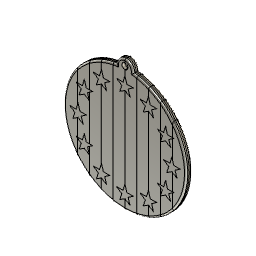
EU-Ohrring-Volt-v4 (Autodesk Fusion 360 design; units mm, degrees)
Autodesk Fusion 360 part; units mm, degrees
sketch "Skizze1" plane through (0, 0, 0) normal (0, 1, 0) x (1, 0, 0)
  circle A0 centre (0, 0) radius 15
  dimension "d1" = 30
  constraint coincident A0.centre origin
  measures "d1" diameter of A0
extrude "Extrusion1" add sketch "Skizze1" along normal blind 1.5 makes body 1
sketch "Skizze2" plane through (0, 0, 0) normal (0, -1, 0) x (1, 0, 0)
  circle A0 centre (0, 0) radius 15
  line L0 (2.7093, -1.1001) -> (1.6674, -1.1001)
  line L1 (1.6674, -1.1001) -> (1.3547, -0.0582)
  line L2 (1.3547, -0.0582) -> (1.0419, -1.1001)
  line L3 (1.0419, -1.1001) -> (0, -1.1001)
  line L4 (0, -1.1001) -> (0.8334, -1.6732)
  line L5 (0.8334, -1.6732) -> (0.5212, -2.6633)
  line L6 (0.5212, -2.6633) -> (1.3547, -2.1421)
  line L7 (1.3547, -2.1421) -> (2.1881, -2.6633)
  line L8 (2.1881, -2.6633) -> (1.8759, -1.6732)
  line L9 (1.8759, -1.6732) -> (2.7093, -1.1001)
extrude "Extrusion2" add sketch "Skizze2" against normal blind 0.6 separate body contours L0 L1 L2 L3 L4 L5 L6 L7 L8 L9 makes body 2
sketch "Skizze3" plane through (0, 0, 0) normal (0, 1, 0) x (1, 0, 0)
  point P0 (0, -11.5)
  point P1 (5.75, -9.9593)
  point P2 (9.9593, -5.75)
  point P3 (11.5, 0)
  point P4 (9.9593, 5.75)
  point P5 (5.75, 9.9593)
  point P6 (0, 11.5)
  point P7 (-5.75, 9.9593)
  point P8 (-9.9593, 5.75)
  point P9 (-11.5, 0)
  point P10 (-9.9593, -5.75)
  point P11 (-5.75, -9.9593)
  dimension "d9" = 360
copy_body "Körper kopieren/einfügen1" bodies 2 makes body 3
move_body "Verschieben2" bodies 3 to x (1, 0, 0) y (0, 1, 0) z (0, 0, 1) at (-1.3547, 0, 12.8608)
copy_body "Körper kopieren/einfügen2" bodies 2 makes body 4
move_body "Verschieben3" bodies 4 to x (1, 0, 0) y (0, 1, 0) z (0, 0, 1) at (4.3953, 0, 11.32)
copy_body "Körper kopieren/einfügen3" bodies 2 makes body 5
move_body "Verschieben4" bodies 5 to x (1, 0, 0) y (0, 1, 0) z (0, 0, 1) at (8.6046, 0, 7.1108)
copy_body "Körper kopieren/einfügen4" bodies 2 makes body 6
move_body "Verschieben5" bodies 6 to x (1, 0, 0) y (0, 1, 0) z (0, 0, 1) at (10.1453, 0, 1.3608)
copy_body "Körper kopieren/einfügen5" bodies 2 makes body 7
move_body "Verschieben6" bodies 7 to x (1, 0, 0) y (0, 1, 0) z (0, 0, 1) at (8.6046, 0, -4.3892)
copy_body "Körper kopieren/einfügen6" bodies 2 makes body 8
move_body "Verschieben7" bodies 8 to x (1, 0, 0) y (0, 1, 0) z (0, 0, 1) at (4.3953, 0, -8.5985)
copy_body "Körper kopieren/einfügen7" bodies 2 makes body 9
move_body "Verschieben8" bodies 9 to x (1, 0, 0) y (0, 1, 0) z (0, 0, 1) at (-1.3547, 0, -10.1392)
copy_body "Körper kopieren/einfügen8" bodies 2 makes body 10
move_body "Verschieben9" bodies 10 to x (1, 0, 0) y (0, 1, 0) z (0, 0, 1) at (-7.1047, 0, -8.5985)
copy_body "Körper kopieren/einfügen9" bodies 2 makes body 11
move_body "Verschieben10" bodies 11 to x (1, 0, 0) y (0, 1, 0) z (0, 0, 1) at (-11.314, 0, -4.3892)
copy_body "Körper kopieren/einfügen10" bodies 2 makes body 12
move_body "Verschieben11" bodies 12 to x (1, 0, 0) y (0, 1, 0) z (0, 0, 1) at (-12.8547, 0, 1.3608)
copy_body "Körper kopieren/einfügen11" bodies 2 makes body 13
move_body "Verschieben12" bodies 13 to x (1, 0, 0) y (0, 1, 0) z (0, 0, 1) at (-11.314, 0, 7.1108)
move_body "Verschieben13" bodies 2 to x (1, 0, 0) y (0, 1, 0) z (0, 0, 1) at (-7.1047, 0, 11.32)
scale "Maßstab1" factors (1.5, 1, 1.5) about (-6.0627, 0, 10.2199) bodies 2
scale "Maßstab2" factors (1.5, 1, 1.5) about (-0.3127, 0, 11.7606) bodies 3
scale "Maßstab3" factors (1.5, 1, 1.5) about (6.0627, 0, 10.2199) bodies 4
scale "Maßstab4" factors (1.5, 1, 1.5) about (10.272, 0, 6.0106) bodies 5
scale "Maßstab5" factors (1.5, 1, 1.5) about (11.8127, 0, 0.2606) bodies 6
scale "Maßstab6" factors (1.5, 1, 1.5) about (10.272, 0, -5.4894) bodies 7
scale "Maßstab7" factors (1.5, 1, 1.5) about (6.0627, 0, -9.6987) bodies 8
scale "Maßstab8" factors (1.5, 1, 1.5) about (-0.3127, 0, -11.2394) bodies 9
scale "Maßstab9" factors (1.5, 1, 1.5) about (-6.0627, 0, -9.6987) bodies 10
scale "Maßstab10" factors (1.5, 1, 1.5) about (-10.272, 0, -5.4894) bodies 11
scale "Maßstab11" factors (1.5, 1, 1.5) about (-11.1873, 0, 0.2606) bodies 12
scale "Maßstab12" factors (1.5, 1, 1.5) about (-10.272, 0, 6.0106) bodies 13
cylinder "Grundkörper Zylinder1" add diameter 4 height 1.5 placed x (1, 0, 0) y (0, 0, -1) z (0, 1, 0) at (0, 0, 15) bodies 1
hole "Bohrung1" at (-0.0089, 0, 15.4827) direction (0, 1, 0) diameter 1.5 depth 3 tip angle 118 bodies 1
fillet "Abrundung1" radius 0.4 1 edges at (0, 0, -15) on bodies 1
fillet "Abrundung2" radius 0.4 1 edges at (0, 0, 17) on bodies 1
fillet "Abrundung3" radius 0.4 1 edges at (0, 1.5, -15) on bodies 1
fillet "Abrundung4" radius 0.4 1 edges at (0, 1.5, 17) on bodies 1
move_body "Verschieben14" bodies 3 to x (1, 0, 0) y (0, 1, 0) z (0, 0, 1) at (-0.1564, 0, 0.1303)
move_body "Verschieben15" bodies 4 to x (1, 0, 0) y (0, 1, 0) z (0, 0, 1) at (0.1564, 0, 0.1303)
move_body "Verschieben16" bodies 6 to x (1, 0, 0) y (0, 1, 0) z (0, 0, 1) at (0.1564, 0, 0.1303)
move_body "Verschieben17" bodies 5 to x (1, 0, 0) y (0, 1, 0) z (0, 0, 1) at (0.1564, 0, 0.1303)
move_body "Verschieben18" bodies 7 to x (1, 0, 0) y (0, 1, 0) z (0, 0, 1) at (0.1564, 0, 0.1303)
move_body "Verschieben19" bodies 8 to x (1, 0, 0) y (0, 1, 0) z (0, 0, 1) at (0.1564, 0, 0.1303)
move_body "Verschieben20" bodies 9 to x (1, 0, 0) y (0, 1, 0) z (0, 0, 1) at (-0.1564, 0, 0.1303)
move_body "Verschieben21" bodies 10 to x (1, 0, 0) y (0, 1, 0) z (0, 0, 1) at (-0.1564, 0, 0.1303)
move_body "Verschieben22" bodies 11 to x (1, 0, 0) y (0, 1, 0) z (0, 0, 1) at (-0.1564, 0, 0.1303)
move_body "Verschieben23" bodies 12 to x (1, 0, 0) y (0, 1, 0) z (0, 0, 1) at (0.1564, 0, 0.1303)
move_body "Verschieben24" bodies 13 to x (1, 0, 0) y (0, 1, 0) z (0, 0, 1) at (-0.1564, 0, 0.1303)
move_body "Verschieben25" bodies 2 to x (1, 0, 0) y (0, 1, 0) z (0, 0, 1) at (-0.1564, 0, 0.1303)
combine "Kombinieren1" operation cut target body 1 tool bodies 2 4 7 6 3 5 10 11 9 12 8 13 keep tools
sketch "Skizze6" plane through (0, 0, 0) normal (0, 1, 0) x (1, 0, 0)
  arc A0 (1.5263, -14.52) -> (-1.5263, -14.52) centre (0, 0) ccw
  line L0 (-14.6, -15) -> (-14.6, 15)
  line L1 (14.6, -15) -> (14.6, 15)
  line L2 (-11.65, -15) -> (-11.65, 15)
  line L3 (-8.7, 15) -> (-8.7, -15)
  line L4 (-5.8, -15) -> (-5.8, 15)
  line L5 (-2.9, -15) -> (-2.9, 15)
  line L6 (0, 15) -> (0, -15)
  line L7 (2.9, -15) -> (2.9, 15)
  line L8 (5.8, -15) -> (5.8, 15)
  line L9 (8.7, -15) -> (8.7, 15)
  line L10 (11.65, -15) -> (11.65, 15)
  dimension "d61" = 14.6
  dimension "d62" = 2.95
  dimension "d63" = 2.95
  dimension "d64" = 2.9
  dimension "d65" = 2.9
  dimension "d66" = 2.9
  dimension "d67" = 2.9
  dimension "d68" = 2.9
  dimension "d69" = 2.9
  dimension "d70" = 2.95
  dimension "d71" = 2.95
  constraint vertical L0
  constraint tangent A0 L0
  constraint vertical L1
  constraint tangent A0 L1
  constraint vertical L2
  constraint parallel L2 L3
  constraint parallel L3 L4
  constraint parallel L3 L5
  constraint parallel L5 L6
  constraint parallel L5 L7
  constraint parallel L7 L8
  constraint parallel L8 L9
  constraint vertical L10
  measures "d61" radius of A0
  measures "d62" distance of L0 L2
  measures "d63" distance of L2 L3
  measures "d64" distance of L3 L4
  measures "d65" distance of L4 L5
  measures "d66" distance of L5 L6
  measures "d67" distance of L6 L7
  measures "d68" distance of L7 L8
  measures "d69" distance of L8 L9
  measures "d70" distance of L9 L10
  measures "d71" distance of L1 L10
ref_plane "Arbeitsebene1" through (-14.6, 0, 0) normal (1, 0, 0) x (0, 0, -1)
ref_plane "Arbeitsebene2" through (-11.65, 0, 0) normal (1, 0, 0) x (0, 0, -1)
ref_plane "Arbeitsebene3" through (-8.7, 0, 0) normal (-1, 0, 0) x (0, 0, 1)
ref_plane "Arbeitsebene4" through (-5.8, 0, 0) normal (1, 0, 0) x (0, 0, -1)
ref_plane "Arbeitsebene5" through (-2.9, 0, 0) normal (1, 0, 0) x (0, 0, -1)
ref_plane "Arbeitsebene6" through (0, 0, 0) normal (-1, 0, 0) x (0, 0, 1)
ref_plane "Arbeitsebene7" through (2.9, 0, 0) normal (1, 0, 0) x (0, 0, -1)
ref_plane "Arbeitsebene8" through (5.8, 0, 0) normal (1, 0, 0) x (0, 0, -1)
ref_plane "Arbeitsebene9" through (8.7, 0, 0) normal (1, 0, 0) x (0, 0, -1)
ref_plane "Arbeitsebene10" through (11.65, 0, 0) normal (1, 0, 0) x (0, 0, -1)
ref_plane "Arbeitsebene11" through (14.6, 0, 0) normal (1, 0, 0) x (0, 0, -1)
split "Teilen1" by plane through (-11.65, 0, 0) normal (1, 0, 0) bodies 1 makes body 14 at (-2.5458, 1.5, -0.3095)
split "Teilen2" by plane through (-8.7, 0, 0) normal (-1, 0, 0) bodies 14 makes body 15 at (-10.3998, 1.5, -2.9333)
split "Teilen3" by plane through (-5.8, 0, 0) normal (1, 0, 0) bodies 14 makes body 16 at (0.4195, 1.5, -2.305)
split "Teilen4" by plane through (-2.9, 0, 0) normal (1, 0, 0) bodies 16 makes body 17 at (0.7735, 1.5, 4.3454)
split "Teilen5" by plane through (0, 0, 0) normal (-1, 0, 0) bodies 17 makes body 18 at (-1.6135, 1.5, -4.9205)
split "Teilen6" by plane through (2.9, 0, 0) normal (1, 0, 0) bodies 17 makes body 19 at (4.8117, 1.5, -3.9242)
split "Teilen7" by plane through (5.8, 0, 0) normal (1, 0, 0) bodies 19 makes body 20 at (7.5048, 1.5, -3.2324)
split "Teilen8" by plane through (8.7, 0, 0) normal (1, 0, 0) bodies 20 makes body 21 at (12.3319, 1.5, 1.7081)
split "Teilen9" by plane through (11.65, 0, 0) normal (1, 0, 0) bodies 21 makes body 22 at (12.6208, 1.5, 0.3495)
sketch "Skizze8" plane through (0, 1.5, 0) normal (0, 1, 0) x (-1, 0, 0)
  line L0 (0, 16.6) -> (0, 16.2326)
  arc A0 (0, 14.7328) -> (0, 16.2326) centre (0.0089, 15.4827) ccw
  line L1 (0, 14.7328) -> (0, -14.6)
  arc A1 (0, -14.6) -> (2.9, -14.3091) centre (0, 0) ccw
  line L2 (2.9, -14.3091) -> (2.9, 14.3091)
  arc A2 (2.9, 14.3091) -> (1.5263, 14.52) centre (0, 0) ccw
  arc A3 (1.5263, 14.52) -> (0, 16.6) centre (0, 15) ccw
  line L3 (8.4482, -1.4987) -> (8.4482, 1.0274)
  line L4 (8.4482, 1.0274) -> (10.3188, 1.0274)
  line L5 (10.3188, 1.0274) -> (10.3188, 2.7193)
  line L6 (10.3188, 2.7193) -> (8.4482, 2.7193)
  line L7 (8.4482, 2.7193) -> (8.4482, 4.9996)
  line L8 (8.4482, 4.9996) -> (6.4136, 4.6772)
  line L9 (6.4136, 4.6772) -> (6.4136, -1.5263)
  spline S0 degree 3 poles (6.4136, -1.5263) (6.4136, -1.9903) (6.4561, -2.4138) (6.5434, -2.7958) knots 0 0 0 0 1 1 1 1
  spline S1 degree 3 poles (6.5434, -2.7958) (6.6296, -3.1778) (6.7818, -3.5034) (7.0009, -3.7715) knots 0 0 0 0 1 1 1 1
  spline S2 degree 3 poles (7.0009, -3.7715) (7.2191, -4.0397) (7.5107, -4.2493) (7.8747, -4.3993) knots 0 0 0 0 1 1 1 1
  spline S3 degree 3 poles (7.8747, -4.3993) (8.2385, -4.5494) (8.6982, -4.6249) (9.2536, -4.6249) knots 0 0 0 0 1 1 1 1
  spline S4 degree 3 poles (9.2536, -4.6249) (9.6909, -4.6249) (10.0591, -4.5887) (10.3591, -4.5153) knots 0 0 0 0 1 1 1 1
  spline S5 degree 3 poles (10.3591, -4.5153) (10.6592, -4.4429) (10.9328, -4.3557) (11.1786, -4.2557) knots 0 0 0 0 1 1 1 1
  line L10 (11.1786, -4.2557) -> (10.8912, -2.6723)
  spline S6 degree 3 poles (10.8912, -2.6723) (10.6996, -2.7458) (10.4889, -2.8022) (10.256, -2.8426) knots 0 0 0 0 1 1 1 1
  spline S7 degree 3 poles (10.256, -2.8426) (10.024, -2.883) (9.7984, -2.9043) (9.5803, -2.9043) knots 0 0 0 0 1 1 1 1
  spline S8 degree 3 poles (9.5803, -2.9043) (9.1248, -2.9043) (8.8227, -2.7766) (8.6727, -2.5223) knots 0 0 0 0 1 1 1 1
  spline S9 degree 3 poles (8.6727, -2.5223) (8.5227, -2.268) (8.4482, -1.9264) (8.4482, -1.4987) knots 0 0 0 0 1 1 1 1
  spline S10 degree 3 poles (-6.1743, -4.461) (-5.7998, -3.6704) (-5.4295, -2.8468) (-5.0656, -1.9913) knots 0 0 0 0 1 1 1 1
  spline S11 degree 3 poles (-5.0656, -1.9913) (-4.7017, -1.1358) (-4.3558, -0.2899) (-4.0281, 0.5475) knots 0 0 0 0 1 1 1 1
  spline S12 degree 3 poles (-4.0281, 0.5475) (-3.7004, 1.385) (-3.3992, 2.1851) (-3.1226, 2.9481) knots 0 0 0 0 1 1 1 1
  spline S13 degree 3 poles (-3.1226, 2.9481) (-2.847, 3.7131) (-2.6033, 4.3963) (-2.3916, 4.9996) knots 0 0 0 0 1 1 1 1
  line L11 (-2.3916, 4.9996) -> (-4.6591, 4.9996)
  spline S14 degree 3 poles (-4.6591, 4.9996) (-4.8368, 4.4484) (-5.0347, 3.8579) (-5.2507, 3.2269) knots 0 0 0 0 1 1 1 1
  spline S15 degree 3 poles (-5.2507, 3.2269) (-5.4678, 2.5948) (-5.688, 1.9649) (-5.9126, 1.3381) knots 0 0 0 0 1 1 1 1
  spline S16 degree 3 poles (-5.9126, 1.3381) (-6.1371, 0.7103) (-6.3552, 0.1102) (-6.5659, -0.4644) knots 0 0 0 0 1 1 1 1
  spline S17 degree 3 poles (-6.5659, -0.4644) (-6.7766, -1.039) (-6.9713, -1.5338) (-7.149, -1.9488) knots 0 0 0 0 1 1 1 1
  spline S18 degree 3 poles (-7.149, -1.9488) (-7.3374, -1.5306) (-7.5353, -1.0347) (-7.7406, -0.4601) knots 0 0 0 0 1 1 1 1
  spline S19 degree 3 poles (-7.7406, -0.4601) (-7.9471, 0.1145) (-8.162, 0.7157) (-8.3865, 1.3424) knots 0 0 0 0 1 1 1 1
  spline S20 degree 3 poles (-8.3865, 1.3424) (-8.6111, 1.9691) (-8.8324, 2.5991) (-9.0494, 3.2301) knots 0 0 0 0 1 1 1 1
  spline S21 degree 3 poles (-9.0494, 3.2301) (-9.2665, 3.8621) (-9.4634, 4.4516) (-9.64, 4.9996) knots 0 0 0 0 1 1 1 1
  line L12 (-9.64, 4.9996) -> (-11.9884, 4.9996)
  spline S22 degree 3 poles (-11.9884, 4.9996) (-11.7873, 4.3995) (-11.5489, 3.7163) (-11.2723, 2.9513) knots 0 0 0 0 1 1 1 1
  spline S23 degree 3 poles (-11.2723, 2.9513) (-10.9956, 2.1862) (-10.6934, 1.386) (-10.3636, 0.5497) knots 0 0 0 0 1 1 1 1
  spline S24 degree 3 poles (-10.3636, 0.5497) (-10.0337, -0.2867) (-9.6858, -1.1326) (-9.3197, -1.9871) knots 0 0 0 0 1 1 1 1
  spline S25 degree 3 poles (-9.3197, -1.9871) (-8.9537, -2.8415) (-8.5823, -3.6662) (-8.2056, -4.461) knots 0 0 0 0 1 1 1 1
  line L13 (-8.2056, -4.461) -> (-6.1743, -4.461)
  line L14 (5.7422, 4.9996) -> (3.7077, 4.6772)
  line L15 (3.7077, 4.6772) -> (3.7077, -4.461)
  line L16 (3.7077, -4.461) -> (5.7422, -4.461)
  line L17 (5.7422, -4.461) -> (5.7422, 4.9996)
  spline S26 degree 3 poles (3.1394, -0.9656) (3.1394, 1.07) (1.4891, 2.7204) (-0.5465, 2.7204) knots 0 0 0 0 1 1 1 1
  spline S27 degree 3 poles (-0.5465, 2.7204) (-1.386, 2.7204) (-2.1596, 2.4394) (-2.7789, 1.9681) knots 0 0 0 0 1 1 1 1
  spline S28 degree 3 poles (-2.7789, 1.9681) (-2.9513, 1.5073) (-3.1321, 1.0349) (-3.3226, 0.5497) knots 0 0 0 0 1 1 1 1
  spline S29 degree 3 poles (-3.3226, 0.5497) (-3.5971, -0.1505) (-3.8834, -0.8581) (-4.1835, -1.571) knots 0 0 0 0 1 1 1 1
  spline S30 degree 3 poles (-4.1835, -1.571) (-3.893, -3.3193) (-2.3756, -4.6515) (-0.5465, -4.6515) knots 0 0 0 0 1 1 1 1
  spline S31 degree 3 poles (-0.5465, -4.6515) (1.4891, -4.6515) (3.1394, -3.0011) (3.1394, -0.9656) knots 0 0 0 0 1 1 1 1
  spline S32 degree 3 poles (1.2944, -0.9656) (1.2944, -1.9733) (0.4772, -2.7905) (-0.5305, -2.7905) knots 0 0 0 0 1 1 1 1
  spline S33 degree 3 poles (-0.5305, -2.7905) (-1.5382, -2.7905) (-2.3554, -1.9733) (-2.3554, -0.9656) knots 0 0 0 0 1 1 1 1
  spline S34 degree 3 poles (-2.3554, -0.9656) (-2.3554, 0.0421) (-1.5382, 0.8593) (-0.5305, 0.8593) knots 0 0 0 0 1 1 1 1
  spline S35 degree 3 poles (-0.5305, 0.8593) (0.4772, 0.8593) (1.2944, 0.0421) (1.2944, -0.9656) knots 0 0 0 0 1 1 1 1
extrude "Extrusion4" cut sketch "Skizze8" against normal blind 0.2 contours L1 L2 S26 S31 S32 S35 | L1 S26 S27 S28 S29 S30 S31 S32 S33 S34 S35 | L3 L4 L5 L6 L7 L8 L9 S0 S1 S2 S3 S4 S5 L10 S6 S7 S8 S9 | S10 S11 S12 S13 L11 S14 S15 S16 S17 S18 S19 S20 S21 L12 S22 S23 S24 S25 L13 | L14 L15 L16 L17 bodies 14 15 16 17 18 19 20 21 22
ref_plane "Arbeitsebene12" through (-1.45, 0.75, 8.4719) normal (0, 1, 0) x (1, 0, 0)
split "Teilen10" by plane through (-1.45, 0.75, 8.4719) normal (0, 1, 0) bodies 1 makes body 23 at (-12.3224, 1.5, 1.7117)
split "Teilen11" by plane through (-1.45, 0.75, 8.4719) normal (0, 1, 0) bodies 15 makes body 24 at (-10.2229, 1.5, 4.7461)
split "Teilen12" by plane through (-1.45, 0.75, 8.4719) normal (0, 1, 0) bodies 14 makes body 25 at (-7.8539, 1.5, 7.1339)
split "Teilen13" by plane through (-1.45, 0.75, 8.4719) normal (0, 1, 0) bodies 16 makes body 26 at (-5.0833, 1.5, -7.4402)
split "Teilen14" by plane through (-1.45, 0.75, 8.4719) normal (0, 1, 0) bodies 17 18 19 20 21 22 makes body 32 at (13.193, 1.5, 4.0905) makes body 31 at (10.4444, 1.5, -3.4124) makes body 30 at (7.7333, 1.5, 5.2013) makes body 29 at (4.8333, 1.5, -6.9525) makes body 28 at (-0.5088, 1.5, 10.6443) makes body 27 at (0.7972, 1.5, 7.4708)
equation "d24 = Sternmaßstab"
equation "d26 = Sternmaßstab"
equation "d27 = Sternmaßstab"
equation "d29 = Sternmaßstab"
equation "d30 = Sternmaßstab"
equation "d32 = Sternmaßstab"
equation "d33 = Sternmaßstab"
equation "d35 = Sternmaßstab"
equation "d36 = Sternmaßstab"
equation "d38 = Sternmaßstab"
equation "d42 = Sternmaßstab"
equation "d44 = Sternmaßstab"
equation "Sternmaßstab = 1.5"
equation "d46 = Sternmaßstab"
equation "d48 = Sternmaßstab"
equation "d49 = Sternmaßstab"
equation "d51 = Sternmaßstab"
equation "d52 = Sternmaßstab"
equation "d54 = Sternmaßstab"
equation "d55 = Sternmaßstab"
equation "d57 = Sternmaßstab"
equation "d58 = Sternmaßstab"
equation "d60 = Sternmaßstab"
named bodies: "Scheibe-1 vorne", "Star 12", "Star1", "Star 1", "Star1 (1)", "Star 2", "Star1 (2)", "Star 3", "Star1 (3)", "Star 4", "Star1 (4)", "Star 5", "Star1 (5)", "Star 6", "Star1 (6)", "Star 7", "Star1 (7)", "Star 8", "Star1 (8)", "Star 9", "Star1 (9)", "Star 10", "Star1 (10)", "Star 11", "Scheibe-3 vorne", "Scheibe-2 vorne", "Scheibe-4 vorne", "Scheibe-6 vorne", "Scheibe-5 vorne", "Scheibe-7 vorne", "Scheibe-8 vorne", "Scheibe-9 vorne", "Scheibe-10 vorne", "Scheibe-1 hinten", "Scheibe-2 hinten", "Scheibe-3 hinten", "Scheibe-4 hinten", "Scheibe-6 hinten", "Scheibe-5 hinten", "Scheibe-7 hinten", "Scheibe-8 hinten", "Scheibe-9 hinten", "Scheibe-10 hinten"
